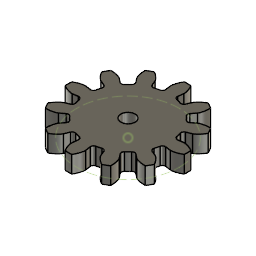
MiniGear (Autodesk Fusion 360 design; units mm, degrees)
description: Spur Gear; Module: 1.5; Num Teeth: 12; Pressure Angle: 14.500000000000002; Backlash: 0.00 mm
Autodesk Fusion 360 part; units mm, degrees
sketch "Base Circle" plane through (0, 0, 0) normal (0, 0, 1) x (1, 0, 0)
  circle A0 centre (0, 0) radius 7.2645
  circle A1 centre (0, 0) radius 1.25
extrude "Extrude1" add sketch "Base Circle" along normal blind 3
sketch "Gear Tooth" plane through (0, 0, 0) normal (0, 0, 1) x (1, 0, 0)
  spline S0 degree 5 poles (8.6323, -1.1852) (8.6375, -1.1859) (8.6479, -1.1872) (8.6636, -1.1886) (8.6845, -1.1897) (8.7108, -1.1899) (8.7371, -1.1892) (8.7635, -1.188) (8.7899, -1.1864) (8.8164, -1.1847) (8.8428, -1.1828) (8.8693, -1.1806) (8.8958, -1.178) (8.9224, -1.1751) (8.949, -1.1717) (8.9756, -1.1679) (9.0022, -1.1638) (9.0288, -1.1594) (9.0554, -1.1547) (9.0821, -1.1498) (9.1087, -1.1447) (9.1354, -1.1393) (9.1621, -1.1337) (9.1887, -1.1278) (9.2154, -1.1217) (9.2421, -1.1153) (9.2688, -1.1086) (9.2955, -1.1017) (9.3222, -1.0946) (9.3488, -1.0873) (9.3755, -1.0797) (9.4022, -1.072) (9.4289, -1.064) (9.4555, -1.0558) (9.4822, -1.0474) (9.5089, -1.0387) (9.5355, -1.0299) (9.5622, -1.0209) (9.5888, -1.0116) (9.6154, -1.0022) (9.642, -0.9925) (9.6686, -0.9827) (9.6952, -0.9727) (9.7218, -0.9624) (9.7483, -0.952) (9.7749, -0.9414) (9.8014, -0.9306) (9.8279, -0.9196) (9.8544, -0.9085) (9.8809, -0.8971) (9.9074, -0.8856) (9.9338, -0.8739) (9.9602, -0.862) (9.9866, -0.8499) (10.013, -0.8376) (10.0394, -0.8252) (10.0657, -0.8126) (10.092, -0.7998) (10.1183, -0.7868) (10.1446, -0.7737) (10.1708, -0.7604) (10.197, -0.7469) (10.2232, -0.7333) (10.2494, -0.7195) (10.2755, -0.7055) (10.3016, -0.6914) (10.3277, -0.677) (10.3538, -0.6626) (10.3798, -0.6479) (10.4058, -0.6331) (10.4317, -0.6182) (10.4525, -0.6061) (10.468, -0.5969) (10.4784, -0.5908) (10.4835, -0.5877) knots 0 0 0 0 0 0 0.01428571 0.02857143 0.04285714 0.05714286 0.07142857 0.08571429 0.1 0.11428571 0.12857143 0.14285714 0.15714286 0.17142857 0.18571429 0.2 0.21428571 0.22857143 0.24285714 0.25714286 0.27142857 0.28571429 0.3 0.31428571 0.32857143 0.34285714 0.35714286 0.37142857 0.38571429 0.4 0.41428571 0.42857143 0.44285714 0.45714286 0.47142857 0.48571429 0.5 0.51428571 0.52857143 0.54285714 0.55714286 0.57142857 0.58571429 0.6 0.61428571 0.62857143 0.64285714 0.65714286 0.67142857 0.68571429 0.7 0.71428571 0.72857143 0.74285714 0.75714286 0.77142857 0.78571429 0.8 0.81428571 0.82857143 0.84285714 0.85714286 0.87142857 0.88571429 0.9 0.91428571 0.92857143 0.94285714 0.95714286 0.97142857 0.98571429 1 1 1 1 1 1
  spline S1 degree 5 poles (8.6323, 1.1852) (8.6375, 1.1859) (8.6479, 1.1872) (8.6636, 1.1886) (8.6845, 1.1897) (8.7108, 1.1899) (8.7371, 1.1892) (8.7635, 1.188) (8.7899, 1.1864) (8.8164, 1.1847) (8.8428, 1.1828) (8.8693, 1.1806) (8.8958, 1.178) (8.9224, 1.1751) (8.949, 1.1717) (8.9756, 1.1679) (9.0022, 1.1638) (9.0288, 1.1594) (9.0554, 1.1547) (9.0821, 1.1498) (9.1087, 1.1447) (9.1354, 1.1393) (9.1621, 1.1337) (9.1887, 1.1278) (9.2154, 1.1217) (9.2421, 1.1153) (9.2688, 1.1086) (9.2955, 1.1017) (9.3222, 1.0946) (9.3488, 1.0873) (9.3755, 1.0797) (9.4022, 1.072) (9.4289, 1.064) (9.4555, 1.0558) (9.4822, 1.0474) (9.5089, 1.0387) (9.5355, 1.0299) (9.5622, 1.0209) (9.5888, 1.0116) (9.6154, 1.0022) (9.642, 0.9925) (9.6686, 0.9827) (9.6952, 0.9727) (9.7218, 0.9624) (9.7483, 0.952) (9.7749, 0.9414) (9.8014, 0.9306) (9.8279, 0.9196) (9.8544, 0.9085) (9.8809, 0.8971) (9.9074, 0.8856) (9.9338, 0.8739) (9.9602, 0.862) (9.9866, 0.8499) (10.013, 0.8376) (10.0394, 0.8252) (10.0657, 0.8126) (10.092, 0.7998) (10.1183, 0.7868) (10.1446, 0.7737) (10.1708, 0.7604) (10.197, 0.7469) (10.2232, 0.7333) (10.2494, 0.7195) (10.2755, 0.7055) (10.3016, 0.6914) (10.3277, 0.677) (10.3538, 0.6626) (10.3798, 0.6479) (10.4058, 0.6331) (10.4317, 0.6182) (10.4525, 0.6061) (10.468, 0.5969) (10.4784, 0.5908) (10.4835, 0.5877) knots 0 0 0 0 0 0 0.01428571 0.02857143 0.04285714 0.05714286 0.07142857 0.08571429 0.1 0.11428571 0.12857143 0.14285714 0.15714286 0.17142857 0.18571429 0.2 0.21428571 0.22857143 0.24285714 0.25714286 0.27142857 0.28571429 0.3 0.31428571 0.32857143 0.34285714 0.35714286 0.37142857 0.38571429 0.4 0.41428571 0.42857143 0.44285714 0.45714286 0.47142857 0.48571429 0.5 0.51428571 0.52857143 0.54285714 0.55714286 0.57142857 0.58571429 0.6 0.61428571 0.62857143 0.64285714 0.65714286 0.67142857 0.68571429 0.7 0.71428571 0.72857143 0.74285714 0.75714286 0.77142857 0.78571429 0.8 0.81428571 0.82857143 0.84285714 0.85714286 0.87142857 0.88571429 0.9 0.91428571 0.92857143 0.94285714 0.95714286 0.97142857 0.98571429 1 1 1 1 1 1
  arc A0 (10.4835, -0.5877) -> (10.4835, 0.5877) centre (0, 0) ccw
  line L0 (7.1871, -0.9868) -> (8.6323, -1.1852)
  line L1 (7.1871, 0.9868) -> (8.6323, 1.1852)
  line L2 (7.1871, -0.9868) -> (7.1871, 0.9868)
  point P0 (8.7608, -1.188)
  point P1 (8.8908, -1.1784)
  point P2 (9.0219, -1.1605)
  point P3 (9.1537, -1.1355)
  point P4 (9.286, -1.1041)
  point P5 (9.4188, -1.067)
  point P6 (9.5519, -1.0243)
  point P7 (9.6852, -0.9764)
  point P8 (9.8186, -0.9235)
  point P9 (9.9519, -0.8657)
  point P10 (10.0852, -0.8031)
  point P11 (10.2183, -0.7358)
  point P12 (10.3511, -0.664)
  point P13 (8.7608, 1.188)
  point P14 (8.8908, 1.1784)
  point P15 (9.0219, 1.1605)
  point P16 (9.1537, 1.1355)
  point P17 (9.286, 1.1041)
  point P18 (9.4188, 1.067)
  point P19 (9.5519, 1.0243)
  point P20 (9.6852, 0.9764)
  point P21 (9.8186, 0.9235)
  point P22 (9.9519, 0.8657)
  point P23 (10.0852, 0.8031)
  point P24 (10.2183, 0.7358)
  point P25 (10.3511, 0.664)
extrude "Extrude2" add sketch "Gear Tooth" along normal blind 3
fillet "Fillet1" radius 0.5 2 edges at (7.197, -0.9881, 1.5) (7.197, 0.9881, 1.5)
pattern_circular "C-Pattern1" count 12 over 360 about axis through (0, 0, 0) along (0, 0, 1) of "Extrude2", "Fillet1"
sketch "Diametrial Pitch Circle" plane through (0, 0, 0) normal (0, 0, 1) x (1, 0, 0)
  circle A0 centre (0, 0) radius 9 construction
named bodies: "Spur Gear (12 teeth)"
